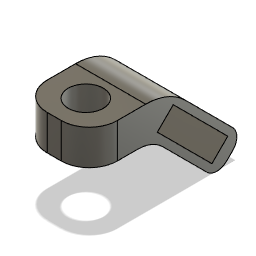
LED_Holder_Back v4 (Autodesk Fusion 360 design; units mm, degrees)
Autodesk Fusion 360 part; units mm, degrees
sketch "Sketch1" plane through (0, 0, 0) normal (1, 0, 0) x (0, 0, -1)
  line L0 (0, 0) -> (9, 0)
  line L1 (9, 0) -> (9, 5)
  line L2 (9, 5) -> (0, 5)
  line L3 (0, 5) -> (0, 0)
  line L4 (9, 0) -> (16.7782, -7.7782)
  line L5 (9, 0) -> (10, 0) construction
  line L6 (16.7782, -7.7782) -> (17.4853, -7.0711)
  line L7 (9, 0) -> (9.7071, 0.7071)
  line L8 (9.7071, 0.7071) -> (17.4853, -7.0711)
  line L9 (17.4853, -7.0711) -> (19.748, -4.8083)
  line L10 (16.7782, -7.7782) -> (18.1924, -9.1924)
  line L11 (19.748, -4.8083) -> (20.4551, -4.1012)
  line L12 (20.4551, -4.1012) -> (21.8693, -5.5154)
  line L13 (21.8693, -5.5154) -> (18.1924, -9.1924)
  line L14 (19.748, -4.8083) -> (11.9698, 2.9698)
  line L15 (11.9698, 2.9698) -> (9.7071, 0.7071)
  line L16 (20.4551, -4.1012) -> (11.3539, 5)
  line L17 (11.3539, 5) -> (9, 5)
  dimension "d1" = 9
  dimension "d2" = 5
  dimension "d3" = 45
  dimension "d4" = 11
  dimension "d5" = 1
  dimension "d6" = 1
  dimension "d7" = 3.2
  dimension "d8" = 2
  dimension "d9" = 1
  dimension "d10" = 2
  constraint horizontal L0
  constraint vertical L1
  constraint horizontal L2
  constraint vertical L3
  constraint coincident L0.start L3.end
  constraint horizontal L5
  constraint perpendicular L4 L6
  constraint perpendicular L4 L7
  constraint perpendicular L8 L9
  constraint perpendicular L6 L10
  constraint parallel L9 L11
  constraint perpendicular L11 L12
  constraint perpendicular L7 L14
  constraint perpendicular L8 L15
  constraint perpendicular L15 L16
  constraint perpendicular L1 L17
  measures "d1" distance of L0.start L0.end
  measures "d2" distance of L0.start L2.end
  measures "d3" angle of L4 L5
  measures "d4" distance of L0.end L4.end
  measures "d5" distance of L4.end L6.end
  measures "d6" distance of L0.end L7.end
  measures "d7" distance of L6.end L9.end
  measures "d8" distance of L4.end L10.end
  measures "d9" distance of L9.end L11.end
  measures "d10" distance of L11.end L12.end
extrude "Extrude1" add sketch "Sketch1" along normal blind 10 contours L0 L1 L2 L3 | L4 L6 L7 L8 | L1 L7 L11 L14 L15 L16 L17 | L6 L9 L10 L11 L12 L13
sketch "Sketch2" plane through (0, 0, 0) normal (0, -1, 0) x (1, 0, 0)
  line L0 (0, 0) -> (0, -9)
  line L1 (0, -9) -> (10, -9)
  line L2 (10, -9) -> (10, 0)
  line L3 (10, 0) -> (0, 0)
  circle A0 centre (5, -4.5) radius 2.5
  line L4 (0, -4.5) -> (5, -4.5)
  dimension "d13" = 5
  constraint midpoint L0 L4.start
  constraint perpendicular L0 L4
  constraint coincident A0.centre L4.end
  measures "d13" diameter of A0
extrude "Extrude2" cut sketch "Sketch2" against normal blind 5 contours A0
hole "Hole1" at (5, 0, -4.5) direction (0, 1, 0) diameter 8 depth 0.5 tip angle 118
fillet "Fillet1" radius 4 2 edges at (10, 2.5, 0) (0, 2.5, 0)
fillet "Fillet2" radius 5 1 edges at (5, 0, -9)
fillet "Fillet3" radius 8 1 edges at (5, 5, -11.3539)
fillet "Fillet4" radius 2 2 edges at (5, -9.1924, -18.1924) (5, -5.5154, -21.8693)
